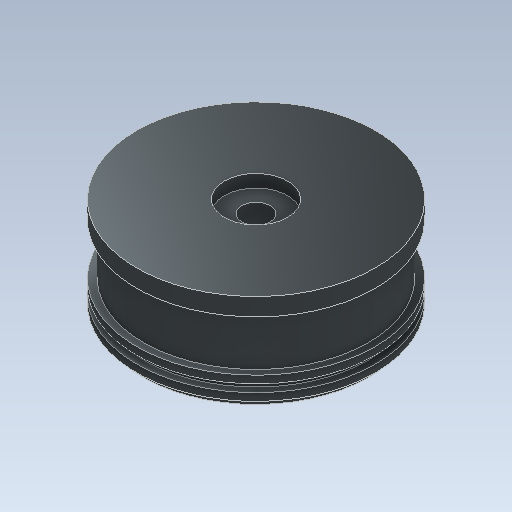
# Autodesk Inventor part: Нижняя часть поршня_CPY
Saved by Autodesk Inventor 2021 (Build 250183000, 183)
## iProperties
Created: 2020-10-24
Part Number: Нижняя часть поршня_CPY
Material: Чугун, серый
Document SubType Name: Modeling
Designer: Тимоха
Mass: 59933.4 g
Surface Area: 6164.49 cm^2
Volume: 8382.29 cm^3
Density: 7.15 g/cm^3
Appearance: Чугун серый
Author: Тимоха
Autodesk Inventor part; units mm, degrees
ref_plane "YZ Plane" through (0, 0, 0) normal (1, 0, 0) x (0, 1, 0)
ref_plane "XZ Plane" through (0, 0, 0) normal (0, 1, 0) x (-1, 0, 0)
ref_plane "XY Plane" through (0, 0, 0) normal (0, 0, 1) x (1, 0, 0)
sketch "Эскиз1" plane through (0, 0, 0) normal (0, 0, 1) x (1, 0, 0)
  line L0 (49.9998, 0) -> (189, 0)
  line L1 (148.768, -39) -> (70.9998, -39)
  line L2 (49.9998, -20) -> (49.9998, 0)
  arc A0 (70.9998, -39) -> (54.9998, -55) centre (70.9998, -55) ccw
  arc A1 (34.9998, -94) -> (24.9998, -84) centre (24.9998, -94) ccw
  line L3 (0, 0) -> (0, 25.6698)
  line L4 (54.9998, -132) -> (54.9998, -55)
  line L5 (189, 0) -> (189, -28)
  line L6 (189, -28) -> (178, -28)
  line L7 (178, -28) -> (178, -108)
  line L8 (178, -108) -> (189, -108)
  line L9 (189, -108) -> (189, -120)
  line L10 (189, -120) -> (178, -120)
  line L11 (178, -120) -> (178, -132)
  line L12 (178, -132) -> (189, -132)
  line L13 (189, -132) -> (189, -144)
  line L14 (189, -144) -> (178, -144)
  line L15 (178, -144) -> (178, -156)
  line L16 (24.9998, -84) -> (22.4998, -84)
  line L17 (22.4998, -84) -> (22.4998, -20)
  line L18 (22.4998, -20) -> (49.9998, -20)
  line L19 (34.9998, -94) -> (34.9998, -156)
  line L20 (34.9998, -156) -> (39.9998, -156)
  line L21 (39.9998, -156) -> (39.9998, -148)
  line L22 (39.9998, -148) -> (54.9998, -148)
  line L23 (54.9998, -148) -> (54.9998, -132)
  line L24 (178, -156) -> (169, -156)
  line L25 (169, -156) -> (169, -148)
  line L26 (169, -148) -> (160, -148)
  line L27 (160, -148) -> (160, -86)
  line L28 (160, -86) -> (164.566, -57.5341)
  arc A2 (164.566, -57.5341) -> (148.768, -39) centre (148.768, -55) ccw
  point P0 (154.5118, -39)
  point P1 (54.9998, -39)
  point P2 (34.9998, -84)
  point P3 (137.0508, -39)
  dimension "d0" = 189
  dimension "d5" = 99.512
  dimension "d9" = 16
  dimension "d11" = 10
  dimension "d29" = 20
  dimension "d30" = 28
  dimension "d31" = 11
  dimension "d32" = 80
  dimension "d34" = 12
  dimension "d35" = 11
  dimension "d36" = 12
  dimension "d37" = 11
  dimension "d38" = 12
  dimension "d39" = 11
  dimension "d40" = 12
  dimension "d43" = 2.5
  dimension "d44" = 64
  dimension "d45" = 15
  dimension "d46" = 8
  dimension "d47" = 5
  dimension "d50" = 9
  dimension "d51" = 9
  dimension "d52" = 16
  constraints: 58 end point, 9 perpendicular, 6 horizontal, 6 point on circle, 6 vertical, 5 point on line, 3 centre point, 3 tangent, 1 collinear
  measures "d0" distance of L3.start L0.end
  measures "d5" distance of point (154.512, -39) point (55, -39)
  measures "d9" radius of A0
  measures "d11" radius of A1
  measures "d29" distance of L2.start L2.end
  measures "d30" distance of L0.end L5.end
  measures "d31" distance of L5.end L6.end
  measures "d32" distance of L6.end L7.end
  measures "d34" distance of L8.end L9.end
  measures "d35" distance of L9.end L10.end
  measures "d36" distance of L10.end L11.end
  measures "d37" distance of L11.end L12.end
  measures "d38" distance of L12.end L13.end
  measures "d39" distance of L13.end L14.end
  measures "d40" distance of L14.end L15.end
  measures "d43" distance of L16.start L16.end
  measures "d44" distance of L16.end L17.end
  measures "d45" distance of L21.end L22.end
  measures "d46" distance of L20.end L21.end
  measures "d47" distance of L19.end L20.end
  measures "d50" distance of L15.end L24.end
  measures "d51" distance of L25.end L26.end
  measures "d52" radius of A2
revolve "Вращение1" add sketch "Эскиз1" angle 360 about axis through (0, 0, 0) along (0, 1, 0)
